Autodesk Inventor part; units mm, degrees
(part 2 of 2)
  spline S149 degree 2 poles (-84.0744, -63.5775) (-83.6641, -63.5775) (-83.2227, -64.1263) (-83.2227, -64.6554) knots 0 0 0 1 2 2 2
  spline S150 degree 2 poles (-84.1423, -64.6809) (-84.1423, -64.463) (-84.3092, -64.2423) (-84.4676, -64.2423) knots 0 0 0 1 2 2 2
  spline S151 degree 2 poles (-84.4676, -64.2423) (-84.6063, -64.2423) (-84.7902, -64.4743) (-84.7902, -64.6583) knots 0 0 0 1 2 2 2
  line L115 (-84.7902, -64.6583) -> (-84.7902, -64.7912)
  spline S152 degree 2 poles (-84.7902, -64.7912) (-84.7902, -64.978) (-84.6233, -65.1987) (-84.4846, -65.1987) knots 0 0 0 1 2 2 2
  spline S153 degree 2 poles (-84.4846, -65.1987) (-84.3205, -65.1987) (-84.1423, -64.9299) (-84.1423, -64.6809) knots 0 0 0 1 2 2 2
  spline S154 degree 2 poles (-82.4588, -66.834) (-82.5862, -66.834) (-82.8776, -66.7887) (-82.9936, -66.7463) knots 0 0 0 1 2 2 2
  line L116 (-82.9936, -66.7463) -> (-82.9936, -66.0644)
  spline S155 degree 2 poles (-82.9936, -66.0644) (-82.9398, -66.104) (-82.7304, -66.1719) (-82.6371, -66.1719) knots 0 0 0 1 2 2 2
  spline S156 degree 2 poles (-82.6371, -66.1719) (-82.3824, -66.1719) (-82.3004, -65.9711) knots 0 0 0 1 1 1
  line L117 (-82.3004, -65.9711) -> (-82.2297, -65.8013)
  line L118 (-82.2297, -65.8013) -> (-83.1407, -63.6312)
  line L119 (-83.1407, -63.6312) -> (-82.1391, -63.6312)
  line L120 (-82.1391, -63.6312) -> (-81.876, -64.6809)
  spline S157 degree 2 poles (-81.876, -64.6809) (-81.7996, -64.9751) (-81.7911, -65.077) knots 0 0 0 1 1 1
  line L121 (-81.7911, -65.077) -> (-81.7826, -65.077)
  spline S158 degree 2 poles (-81.7826, -65.077) (-81.777, -65.0289) (-81.7543, -64.9157) (-81.4346, -63.6312) knots 0 0 0 1 2 2 2
  line L122 (-81.4346, -63.6312) -> (-80.5547, -63.6312)
  line L123 (-80.5547, -63.6312) -> (-81.3554, -65.872)
  spline S159 degree 2 poles (-81.3554, -65.872) (-81.5365, -66.387) (-82.0712, -66.834) (-82.4588, -66.834) knots 0 0 0 1 2 2 2
  spline S160 degree 2 poles (-79.3947, -65.4307) (-79.3947, -65.6259) (-79.6663, -65.8635) (-79.9068, -65.8635) knots 0 0 0 1 2 2 2
  spline S161 degree 2 poles (-79.9068, -65.8635) (-80.1275, -65.8635) (-80.4048, -65.6146) (-80.4048, -65.4307) knots 0 0 0 1 2 2 2
  spline S162 degree 2 poles (-80.4048, -65.4307) (-80.4048, -65.2439) (-80.1303, -65.0119) (-79.8983, -65.0119) knots 0 0 0 1 2 2 2
  spline S163 degree 2 poles (-79.8983, -65.0119) (-79.672, -65.0119) (-79.3947, -65.2439) (-79.3947, -65.4307) knots 0 0 0 1 2 2 2
  spline S164 degree 2 poles (-79.3947, -64.05) (-79.3947, -64.2452) (-79.6691, -64.48) (-79.9068, -64.48) knots 0 0 0 1 2 2 2
  spline S165 degree 2 poles (-79.9068, -64.48) (-80.1246, -64.48) (-80.4048, -64.2339) (-80.4048, -64.05) knots 0 0 0 1 2 2 2
  spline S166 degree 2 poles (-80.4048, -64.05) (-80.4048, -63.8632) (-80.1303, -63.6312) (-79.8983, -63.6312) knots 0 0 0 1 2 2 2
  spline S167 degree 2 poles (-79.8983, -63.6312) (-79.672, -63.6312) (-79.3947, -63.8632) (-79.3947, -64.05) knots 0 0 0 1 2 2 2
  spline S168 degree 2 poles (-137.9162, -70.7081) (-137.9162, -70.8722) (-138.086, -71.1636) (-138.3774, -71.3305) (-138.5387, -71.3305) knots 0 0 0 1 2 3 3 3
  spline S169 degree 2 poles (-138.5387, -71.3305) (-138.7905, -71.3305) (-139.1526, -70.9684) (-139.1526, -70.7081) knots 0 0 0 1 2 2 2
  spline S170 degree 2 poles (-139.1526, -70.7081) (-139.1526, -70.4563) (-138.7961, -70.0941) (-138.5387, -70.0941) knots 0 0 0 1 2 2 2
  spline S171 degree 2 poles (-138.5387, -70.0941) (-138.2755, -70.0941) (-137.9162, -70.4619) (-137.9162, -70.7081) knots 0 0 0 1 2 2 2
  line L124 (-128.1268, -71.7464) -> (-128.2598, -71.1862)
  line L125 (-128.2598, -71.1862) -> (-129.1708, -71.1862)
  line L126 (-129.1708, -71.1862) -> (-129.3151, -71.7464)
  line L127 (-129.3151, -71.7464) -> (-130.3082, -71.7464)
  line L128 (-130.3082, -71.7464) -> (-129.2585, -68.6964)
  line L129 (-129.2585, -68.6964) -> (-128.1183, -68.6964)
  line L130 (-128.1183, -68.6964) -> (-127.128, -71.7464)
  line L131 (-127.128, -71.7464) -> (-128.1268, -71.7464)
  line L132 (-128.704, -69.3613) -> (-128.7238, -69.3613)
  spline S172 degree 2 poles (-128.7238, -69.3613) (-128.7294, -69.4123) (-128.7804, -69.6471) (-129.0124, -70.5327) knots 0 0 0 1 2 2 2
  line L133 (-129.0124, -70.5327) -> (-128.4295, -70.5327)
  line L134 (-128.4295, -70.5327) -> (-128.6417, -69.7037)
  spline S173 degree 2 poles (-128.6417, -69.7037) (-128.687, -69.5198) (-128.704, -69.3613) knots 0 0 0 1 1 1
  line L135 (-126.8536, -71.7464) -> (-126.8536, -68.521)
  line L136 (-126.8536, -68.521) -> (-125.9482, -68.521)
  line L137 (-125.9482, -68.521) -> (-125.9482, -71.7464)
  line L138 (-125.9482, -71.7464) -> (-126.8536, -71.7464)
  spline S174 degree 2 poles (-123.8347, -69.1803) (-123.9762, -69.1322) (-124.095, -69.1322) knots 0 0 0 1 1 1
  spline S175 degree 2 poles (-124.095, -69.1322) (-124.2478, -69.1322) (-124.3921, -69.2878) (-124.3921, -69.4179) knots 0 0 0 1 2 2 2
  line L139 (-124.3921, -69.4179) -> (-124.3921, -69.5679)
  line L140 (-124.3921, -69.5679) -> (-123.8885, -69.5679)
  line L141 (-123.8885, -69.5679) -> (-123.8885, -70.196)
  line L142 (-123.8885, -70.196) -> (-124.3921, -70.196)
  line L143 (-124.3921, -70.196) -> (-124.3921, -71.7464)
  line L144 (-124.3921, -71.7464) -> (-125.2975, -71.7464)
  line L145 (-125.2975, -71.7464) -> (-125.2975, -70.196)
  line L146 (-125.2975, -70.196) -> (-125.6625, -70.196)
  line L147 (-125.6625, -70.196) -> (-125.6625, -69.5679)
  line L148 (-125.6625, -69.5679) -> (-125.2975, -69.5679)
  line L149 (-125.2975, -69.5679) -> (-125.2975, -69.367)
  spline S176 degree 2 poles (-125.2975, -69.367) (-125.2975, -69.101) (-125.0513, -68.6964) (-124.5817, -68.4701) (-124.245, -68.4701) knots 0 0 0 1 2 3 3 3
  spline S177 degree 2 poles (-124.245, -68.4701) (-124.0016, -68.4701) (-123.8347, -68.5182) knots 0 0 0 1 1 1
  line L150 (-123.8347, -68.5182) -> (-123.8347, -69.1803)
  line L151 (-122.4257, -71.7464) -> (-122.4257, -71.4154)
  line L152 (-122.4257, -71.4154) -> (-122.4342, -71.4154)
  spline S178 degree 2 poles (-122.4342, -71.4154) (-122.6521, -71.8002) (-123.0991, -71.8002) knots 0 0 0 1 1 1
  spline S179 degree 2 poles (-123.0991, -71.8002) (-123.4075, -71.8002) (-123.7555, -71.4352) (-123.7555, -71.1268) knots 0 0 0 1 2 2 2
  spline S180 degree 2 poles (-123.7555, -71.1268) (-123.7555, -70.4846) (-122.9661, -70.3827) knots 0 0 0 1 1 1
  line L153 (-122.9661, -70.3827) -> (-122.4257, -70.312)
  spline S181 degree 2 poles (-122.4257, -70.312) (-122.4257, -70.2045) (-122.6181, -70.0687) (-122.7794, -70.0687) knots 0 0 0 1 2 2 2
  spline S182 degree 2 poles (-122.7794, -70.0687) (-123.1444, -70.0687) (-123.5518, -70.278) knots 0 0 0 1 1 1
  line L154 (-123.5518, -70.278) -> (-123.5518, -69.6895)
  spline S183 degree 2 poles (-123.5518, -69.6895) (-123.3764, -69.6131) (-122.8416, -69.5141) (-122.6521, -69.5141) knots 0 0 0 1 2 2 2
  spline S184 degree 2 poles (-122.6521, -69.5141) (-122.0975, -69.5141) (-121.5967, -69.9894) (-121.5967, -70.544) knots 0 0 0 1 2 2 2
  line L155 (-121.5967, -70.544) -> (-121.5967, -71.7464)
  line L156 (-121.5967, -71.7464) -> (-122.4257, -71.7464)
  spline S185 degree 2 poles (-122.9633, -71.0052) (-122.9633, -71.0929) (-122.8501, -71.2089) (-122.7454, -71.2089) knots 0 0 0 1 2 2 2
  spline S186 degree 2 poles (-122.7454, -71.2089) (-122.604, -71.2089) (-122.4257, -70.9967) (-122.4257, -70.8298) knots 0 0 0 1 2 2 2
  line L157 (-122.4257, -70.8298) -> (-122.4257, -70.7477)
  line L158 (-122.4257, -70.7477) -> (-122.7341, -70.7901)
  spline S187 degree 2 poles (-122.7341, -70.7901) (-122.9633, -70.8298) (-122.9633, -71.0052) knots 0 0 0 1 1 1
  line L159 (-119.7775, -71.7464) -> (-119.7775, -70.5581)
  spline S188 degree 2 poles (-119.7775, -70.5581) (-119.7775, -70.3544) (-119.8991, -70.179) (-120.0349, -70.179) knots 0 0 0 1 2 2 2
  spline S189 degree 2 poles (-120.0349, -70.179) (-120.1509, -70.179) (-120.2839, -70.3629) (-120.2839, -70.5044) knots 0 0 0 1 2 2 2
  line L160 (-120.2839, -70.5044) -> (-120.2839, -71.7464)
  line L161 (-120.2839, -71.7464) -> (-121.1893, -71.7464)
  line L162 (-121.1893, -71.7464) -> (-121.1893, -69.5679)
  line L163 (-121.1893, -69.5679) -> (-120.2839, -69.5679)
  line L164 (-120.2839, -69.5679) -> (-120.2839, -69.9074)
  line L165 (-120.2839, -69.9074) -> (-120.2754, -69.9074)
  spline S190 degree 2 poles (-120.2754, -69.9074) (-120.1679, -69.7207) (-119.8001, -69.5141) (-119.5851, -69.5141) knots 0 0 0 1 2 2 2
  spline S191 degree 2 poles (-119.5851, -69.5141) (-118.8721, -69.5141) (-118.8721, -70.4167) knots 0 0 0 1 1 1
  line L166 (-118.8721, -70.4167) -> (-118.8721, -71.7464)
  line L167 (-118.8721, -71.7464) -> (-119.7775, -71.7464)
  spline S192 degree 2 poles (-116.04, -70.6176) (-116.04, -71.1693) (-116.7048, -71.8002) (-117.3018, -71.8002) knots 0 0 0 1 2 2 2
  spline S193 degree 2 poles (-117.3018, -71.8002) (-117.896, -71.8002) (-118.558, -71.1862) (-118.558, -70.643) knots 0 0 0 1 2 2 2
  spline S194 degree 2 poles (-118.558, -70.643) (-118.558, -70.2978) (-118.2468, -69.7857) (-117.6725, -69.5141) (-117.299, -69.5141) knots 0 0 0 1 2 3 3 3
  spline S195 degree 2 poles (-117.299, -69.5141) (-116.9114, -69.5141) (-116.3427, -69.7999) (-116.04, -70.3063) (-116.04, -70.6176) knots 0 0 0 1 2 3 3 3
  spline S196 degree 2 poles (-116.9595, -70.6232) (-116.9595, -70.179) (-117.299, -70.179) knots 0 0 0 1 1 1
  spline S197 degree 2 poles (-117.299, -70.179) (-117.6385, -70.179) (-117.6385, -70.643) knots 0 0 0 1 1 1
  spline S198 degree 2 poles (-117.6385, -70.643) (-117.6385, -71.1353) (-117.2933, -71.1353) knots 0 0 0 1 1 1
  spline S199 degree 2 poles (-117.2933, -71.1353) (-116.9595, -71.1353) (-116.9595, -70.6232) knots 0 0 0 1 1 1
  line L168 (-114.4074, -71.7464) -> (-114.4074, -68.6964)
  line L169 (-114.4074, -68.6964) -> (-112.509, -68.6964)
  line L170 (-112.509, -68.6964) -> (-112.509, -69.4151)
  line L171 (-112.509, -69.4151) -> (-113.4879, -69.4151)
  line L172 (-113.4879, -69.4151) -> (-113.4879, -69.8593)
  line L173 (-113.4879, -69.8593) -> (-112.5684, -69.8593)
  line L174 (-112.5684, -69.8593) -> (-112.5684, -70.5779)
  line L175 (-112.5684, -70.5779) -> (-113.4879, -70.5779)
  line L176 (-113.4879, -70.5779) -> (-113.4879, -71.0278)
  line L177 (-113.4879, -71.0278) -> (-112.4382, -71.0278)
  line L178 (-112.4382, -71.0278) -> (-112.4382, -71.7464)
  line L179 (-112.4382, -71.7464) -> (-114.4074, -71.7464)
  line L180 (-109.2609, -71.7464) -> (-109.2609, -70.4902)
  spline S200 degree 2 poles (-109.2609, -70.4902) (-109.2609, -70.3346) (-109.3741, -70.179) (-109.5014, -70.179) knots 0 0 0 1 2 2 2
  spline S201 degree 2 poles (-109.5014, -70.179) (-109.6259, -70.179) (-109.7674, -70.3686) (-109.7674, -70.5355) knots 0 0 0 1 2 2 2
  line L181 (-109.7674, -70.5355) -> (-109.7674, -71.7464)
  line L182 (-109.7674, -71.7464) -> (-110.6727, -71.7464)
  line L183 (-110.6727, -71.7464) -> (-110.6727, -70.5129)
  spline S202 degree 2 poles (-110.6727, -70.5129) (-110.6727, -70.179) (-110.8991, -70.179) knots 0 0 0 1 1 1
  spline S203 degree 2 poles (-110.8991, -70.179) (-111.0377, -70.179) (-111.1792, -70.3714) (-111.1792, -70.5525) knots 0 0 0 1 2 2 2
  line L184 (-111.1792, -70.5525) -> (-111.1792, -71.7464)
  line L185 (-111.1792, -71.7464) -> (-112.0846, -71.7464)
  line L186 (-112.0846, -71.7464) -> (-112.0846, -69.5679)
  line L187 (-112.0846, -69.5679) -> (-111.1792, -69.5679)
  line L188 (-111.1792, -69.5679) -> (-111.1792, -69.9131)
  line L189 (-111.1792, -69.9131) -> (-111.1707, -69.9131)
  spline S204 degree 2 poles (-111.1707, -69.9131) (-111.1198, -69.8225) (-110.8963, -69.6301) (-110.6162, -69.5141) (-110.4521, -69.5141) knots 0 0 0 1 2 3 3 3
  spline S205 degree 2 poles (-110.4521, -69.5141) (-110.2201, -69.5141) (-109.9032, -69.698) (-109.7985, -69.8961) knots 0 0 0 1 2 2 2
  spline S206 degree 2 poles (-109.7985, -69.8961) (-109.6825, -69.7122) (-109.2977, -69.5141) (-109.0657, -69.5141) knots 0 0 0 1 2 2 2
  spline S207 degree 2 poles (-109.0657, -69.5141) (-108.7205, -69.5141) (-108.3555, -69.9612) (-108.3555, -70.3827) knots 0 0 0 1 2 2 2
  line L190 (-108.3555, -70.3827) -> (-108.3555, -71.7464)
  line L191 (-108.3555, -71.7464) -> (-109.2609, -71.7464)
  line L192 (-106.7372, -71.7464) -> (-106.7372, -71.4154)
  line L193 (-106.7372, -71.4154) -> (-106.7457, -71.4154)
  spline S208 degree 2 poles (-106.7457, -71.4154) (-106.9635, -71.8002) (-107.4106, -71.8002) knots 0 0 0 1 1 1
  spline S209 degree 2 poles (-107.4106, -71.8002) (-107.7189, -71.8002) (-108.067, -71.4352) (-108.067, -71.1268) knots 0 0 0 1 2 2 2
  spline S210 degree 2 poles (-108.067, -71.1268) (-108.067, -70.4846) (-107.2776, -70.3827) knots 0 0 0 1 1 1
  line L194 (-107.2776, -70.3827) -> (-106.7372, -70.312)
  spline S211 degree 2 poles (-106.7372, -70.312) (-106.7372, -70.2045) (-106.9296, -70.0687) (-107.0908, -70.0687) knots 0 0 0 1 2 2 2
  spline S212 degree 2 poles (-107.0908, -70.0687) (-107.4558, -70.0687) (-107.8632, -70.278) knots 0 0 0 1 1 1
  line L195 (-107.8632, -70.278) -> (-107.8632, -69.6895)
  spline S213 degree 2 poles (-107.8632, -69.6895) (-107.6878, -69.6131) (-107.1531, -69.5141) (-106.9635, -69.5141) knots 0 0 0 1 2 2 2
  spline S214 degree 2 poles (-106.9635, -69.5141) (-106.409, -69.5141) (-105.9082, -69.9894) (-105.9082, -70.544) knots 0 0 0 1 2 2 2
  line L196 (-105.9082, -70.544) -> (-105.9082, -71.7464)
  line L197 (-105.9082, -71.7464) -> (-106.7372, -71.7464)
  spline S215 degree 2 poles (-107.2747, -71.0052) (-107.2747, -71.0929) (-107.1616, -71.2089) (-107.0569, -71.2089) knots 0 0 0 1 2 2 2
  spline S216 degree 2 poles (-107.0569, -71.2089) (-106.9154, -71.2089) (-106.7372, -70.9967) (-106.7372, -70.8298) knots 0 0 0 1 2 2 2
  line L198 (-106.7372, -70.8298) -> (-106.7372, -70.7477)
  line L199 (-106.7372, -70.7477) -> (-107.0456, -70.7901)
  spline S217 degree 2 poles (-107.0456, -70.7901) (-107.2747, -70.8298) (-107.2747, -71.0052) knots 0 0 0 1 1 1
  line L200 (-104.0889, -71.7464) -> (-104.0889, -70.5581)
  spline S218 degree 2 poles (-104.0889, -70.5581) (-104.0889, -70.3544) (-104.2106, -70.179) (-104.3464, -70.179) knots 0 0 0 1 2 2 2
  spline S219 degree 2 poles (-104.3464, -70.179) (-104.4624, -70.179) (-104.5954, -70.3629) (-104.5954, -70.5044) knots 0 0 0 1 2 2 2
  line L201 (-104.5954, -70.5044) -> (-104.5954, -71.7464)
  line L202 (-104.5954, -71.7464) -> (-105.5008, -71.7464)
  line L203 (-105.5008, -71.7464) -> (-105.5008, -69.5679)
  line L204 (-105.5008, -69.5679) -> (-104.5954, -69.5679)
  line L205 (-104.5954, -69.5679) -> (-104.5954, -69.9074)
  line L206 (-104.5954, -69.9074) -> (-104.5869, -69.9074)
  spline S220 degree 2 poles (-104.5869, -69.9074) (-104.4794, -69.7207) (-104.1116, -69.5141) (-103.8965, -69.5141) knots 0 0 0 1 2 2 2
  spline S221 degree 2 poles (-103.8965, -69.5141) (-103.1836, -69.5141) (-103.1836, -70.4167) knots 0 0 0 1 1 1
  line L207 (-103.1836, -70.4167) -> (-103.1836, -71.7464)
  line L208 (-103.1836, -71.7464) -> (-104.0889, -71.7464)
  line L209 (-101.3869, -71.7464) -> (-101.3869, -71.4098)
  line L210 (-101.3869, -71.4098) -> (-101.3954, -71.4098)
  spline S222 degree 2 poles (-101.3954, -71.4098) (-101.5086, -71.5654) (-101.6897, -71.7097) (-101.916, -71.8002) (-102.066, -71.8002) knots 0 0 0 1 2 3 3 3
  spline S223 degree 2 poles (-102.066, -71.8002) (-102.4253, -71.8002) (-102.7988, -71.3362) (-102.7988, -70.8835) knots 0 0 0 1 2 2 2
  line L211 (-102.7988, -70.8835) -> (-102.7988, -69.5679)
  line L212 (-102.7988, -69.5679) -> (-101.8934, -69.5679)
  line L213 (-101.8934, -69.5679) -> (-101.8934, -70.8128)
  spline S224 degree 2 poles (-101.8934, -70.8128) (-101.8934, -71.1353) (-101.6529, -71.1353) knots 0 0 0 1 1 1
  spline S225 degree 2 poles (-101.6529, -71.1353) (-101.5199, -71.1353) (-101.3869, -70.9599) (-101.3869, -70.8015) knots 0 0 0 1 2 2 2
  line L214 (-101.3869, -70.8015) -> (-101.3869, -69.5679)
  line L215 (-101.3869, -69.5679) -> (-100.4816, -69.5679)
  line L216 (-100.4816, -69.5679) -> (-100.4816, -71.7464)
  line L217 (-100.4816, -71.7464) -> (-101.3869, -71.7464)
  spline S226 degree 2 poles (-99.265, -70.9146) (-99.2423, -71.0561) (-98.965, -71.2145) (-98.7387, -71.2145) knots 0 0 0 1 2 2 2
  spline S227 degree 2 poles (-98.7387, -71.2145) (-98.4218, -71.2145) (-98.1389, -71.0929) knots 0 0 0 1 1 1
  line L218 (-98.1389, -71.0929) -> (-98.1389, -71.6672)
  spline S228 degree 2 poles (-98.1389, -71.6672) (-98.4671, -71.8002) (-98.9396, -71.8002) knots 0 0 0 1 1 1
  spline S229 degree 2 poles (-98.9396, -71.8002) (-99.5083, -71.8002) (-100.142, -71.2174) (-100.142, -70.7053) knots 0 0 0 1 2 2 2
  spline S230 degree 2 poles (-100.142, -70.7053) (-100.142, -70.3544) (-99.8648, -69.8197) (-99.3187, -69.5141) (-98.9877, -69.5141) knots 0 0 0 1 2 3 3 3
  spline S231 degree 2 poles (-98.9877, -69.5141) (-98.651, -69.5141) (-98.17, -69.7772) (-97.921, -70.2554) (-97.921, -70.5751) knots 0 0 0 1 2 3 3 3
  line L219 (-97.921, -70.5751) -> (-97.921, -70.9146)
  line L220 (-97.921, -70.9146) -> (-99.265, -70.9146)
  spline S232 degree 2 poles (-98.7217, -70.4393) (-98.7217, -70.063) (-98.9905, -70.063) knots 0 0 0 1 1 1
  spline S233 degree 2 poles (-98.9905, -70.063) (-99.1037, -70.063) (-99.2565, -70.2695) (-99.2706, -70.4393) knots 0 0 0 1 2 2 2
  line L221 (-99.2706, -70.4393) -> (-98.7217, -70.4393)
  line L222 (-97.607, -71.7464) -> (-97.607, -68.521)
  line L223 (-97.607, -68.521) -> (-96.7016, -68.521)
  line L224 (-96.7016, -68.521) -> (-96.7016, -71.7464)
  line L225 (-96.7016, -71.7464) -> (-97.607, -71.7464)
  spline S234 degree 2 poles (-95.485, -70.9146) (-95.4624, -71.0561) (-95.1851, -71.2145) (-94.9587, -71.2145) knots 0 0 0 1 2 2 2
  spline S235 degree 2 poles (-94.9587, -71.2145) (-94.6419, -71.2145) (-94.3589, -71.0929) knots 0 0 0 1 1 1
  line L226 (-94.3589, -71.0929) -> (-94.3589, -71.6672)
  spline S236 degree 2 poles (-94.3589, -71.6672) (-94.6871, -71.8002) (-95.1596, -71.8002) knots 0 0 0 1 1 1
  spline S237 degree 2 poles (-95.1596, -71.8002) (-95.7283, -71.8002) (-96.3621, -71.2174) (-96.3621, -70.7053) knots 0 0 0 1 2 2 2
  spline S238 degree 2 poles (-96.3621, -70.7053) (-96.3621, -70.3544) (-96.0848, -69.8197) (-95.5388, -69.5141) (-95.2077, -69.5141) knots 0 0 0 1 2 3 3 3
  spline S239 degree 2 poles (-95.2077, -69.5141) (-94.871, -69.5141) (-94.39, -69.7772) (-94.1411, -70.2554) (-94.1411, -70.5751) knots 0 0 0 1 2 3 3 3
  line L227 (-94.1411, -70.5751) -> (-94.1411, -70.9146)
  line L228 (-94.1411, -70.9146) -> (-95.485, -70.9146)
  spline S240 degree 2 poles (-94.9418, -70.4393) (-94.9418, -70.063) (-95.2106, -70.063) knots 0 0 0 1 1 1
  spline S241 degree 2 poles (-95.2106, -70.063) (-95.3237, -70.063) (-95.4765, -70.2695) (-95.4907, -70.4393) knots 0 0 0 1 2 2 2
  line L229 (-95.4907, -70.4393) -> (-94.9418, -70.4393)
  point P0 (0, 0)
  constraints: 3 other
extrude "Estrusione5" cut sketch "Schizzo6" against normal blind 1
